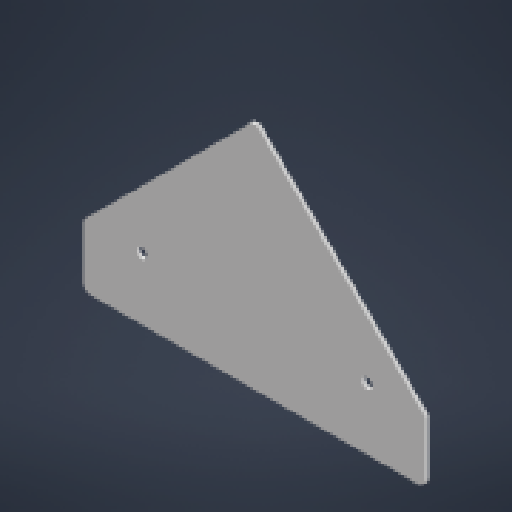
# Autodesk Inventor part: alignernew
Saved by Autodesk Inventor 2026.1 (Build 301233000, 233)
## iProperties
Created: 2026-01-08
Part Number: alignernew
Material: Generic
Document SubType Name: Modeling
Designer: roejo
Density: 1 g/cm^3
Appearance: Default
Author: roejo
Autodesk Inventor part; units mm, degrees
ref_plane "YZ Plane" through (0, 0, 0) normal (1, 0, 0) x (0, 1, 0)
ref_plane "XZ Plane" through (0, 0, 0) normal (0, 1, 0) x (-1, 0, 0)
ref_plane "XY Plane" through (0, 0, 0) normal (0, 0, 1) x (1, 0, 0)
sketch "Sketch1" plane through (0, 0, 0) normal (0, 0, 1) x (1, 0, 0)
  arc A0 (145.923, -27.051) -> (149.098, -23.876) centre (145.923, -23.876) ccw
  line L0 (149.098, -1.3151) -> (149.098, -23.876)
  line L1 (0, -23.876) -> (0, -1.3151)
  line L2 (148.1681, 0.9299) -> (76.7941, 72.3039)
  line L3 (0.9299, 0.9299) -> (72.3039, 72.3039)
  circle A1 centre (25.4, 0) radius 2.2098
  circle A2 centre (123.698, 0) radius 2.2098
  arc A3 (0, -23.876) -> (3.175, -27.051) centre (3.175, -23.876) ccw
  arc A4 (76.7941, 72.3039) -> (72.3039, 72.3039) centre (74.549, 70.0589) ccw
  arc A5 (0.9299, 0.9299) -> (0, -1.3151) centre (3.175, -1.3151) ccw
  arc A6 (149.098, -1.3151) -> (148.1681, 0.9299) centre (145.923, -1.3151) ccw
  line L4 (74.549, 73.2339) -> (74.549, -27.051)
  line L5 (145.923, -27.051) -> (3.175, -27.051)
  point P0 (0, 0)
  point P1 (76.7941, 72.3039)
  point P2 (0, -1.3151)
  point P3 (74.549, 23.0914)
  point P4 (3.175, -27.051)
  constraints: 12 end point, 11 point on circle, 7 centre point, 1 midpoint
extrude "Extrusion1" add sketch "Sketch1" along normal blind 1.5875
body "Solid1"
